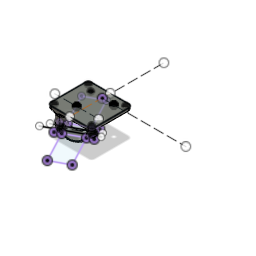
t-echo bracket v3 (Autodesk Fusion 360 design; units mm, degrees)
Autodesk Fusion 360 part; units mm, degrees
note: some values were not read from the file. Chosen so that the rebuilt part matches the saved one: a direction. Set by a fixed rule: which sketch regions a step uses.
sketch "plate" plane through (0, 0, 0) normal (0, 1, 0) x (1, 0, 0)
  line L0 (0, 0) -> (101.1488, 0) construction
  line L1 (0, 0) -> (0, 74.5682) construction
  circle A0 centre (14, 0) radius 1.6
  circle A1 centre (-14, 0) radius 1.6
  line L2 (26, 6) -> (26, -35)
  line L3 (-27, 6) -> (-27, -35)
  line L4 (-23, 10) -> (22, 10)
  line L5 (22, -39) -> (-23, -39)
  arc A2 (-23, 10) -> (-27, 6) centre (-23, 6) ccw
  arc A3 (26, 6) -> (22, 10) centre (22, 6) ccw
  arc A4 (22, -39) -> (26, -35) centre (22, -35) ccw
  arc A5 (-27, -35) -> (-23, -39) centre (-23, -35) ccw
  line L6 (19.5, -24) -> (-33.5, -24) construction
  line L7 (-0.5, -39) -> (-0.5, 10) construction
  point P0 (-7, -24)
  dimension "d1" = 3.2
  dimension "d2" = 14
  dimension "d3" = 12
  dimension "d4" = 53
  dimension "d5" = 10
  dimension "d6" = 39
  dimension "d7" = 4
  dimension "d35" = 20
  dimension "d36" = 15
  constraint coincident L0.start L1.start
  constraint horizontal L0
  constraint perpendicular L0 L1
  constraint coincident L0 A0.centre
  constraint symmetric L1 A0 A1
  constraint vertical L2
  constraint parallel L2 L3
  constraint horizontal L4
  constraint perpendicular L3 L5
  constraint tangent L4 A2
  constraint tangent L3 A2
  constraint tangent L4 A3
  constraint tangent L2 A3
  constraint equal A2 A3
  constraint tangent L2 A4
  constraint tangent L5 A4
  constraint equal A2 A4
  constraint tangent L3 A5
  constraint tangent L5 A5
  constraint equal A2 A5
  constraint midpoint L6 P0
  measures "d1" diameter of A0
  measures "d2" distance of L1 A0.centre
  measures "d3" distance of A0.centre L2
  measures "d4" distance of L2 L3
  measures "d5" distance of A0.centre L4
  measures "d6" distance of A0.centre L5
  measures "d7" radius of A2
  measures "d35" distance of L3 P0
  measures "d36" distance of L5 L6
extrude "Extrude1" add sketch "plate" against normal blind 5 makes body 1
ref_plane "WorkPlane1" through (-6.8327, -2.5, 24.0349) normal (0.469472, 0, 0.882948) x (0, 1, 0)
sketch "bracket" plane through (8.457, 0, 15.9053) normal (0.469472, 0, 0.882948) x (0, 1, 0)
  line L0 (-6, 17.3166) -> (1, 17.3166) construction
  line L1 (-5, 15.6131) -> (-5, -24.1196) construction
  line L2 (-6, 17.3166) -> (-35.5255, 17.3166) construction
  circle A0 centre (-19.15, 17.3166) radius 11.15
  circle A1 centre (-19.15, 17.3166) radius 14.15
  line L3 (-20.15, -0.6834) -> (-18.15, -0.6834)
  line L4 (-18.15, -0.6834) -> (-18.15, 35.3166)
  line L5 (-18.15, 35.3166) -> (-20.15, 35.3166)
  line L6 (-20.15, 35.3166) -> (-20.15, -0.6834)
  line L7 (-20.15, -0.6834) -> (-18.15, 35.3166) construction
  line L8 (-18.15, -0.6834) -> (-20.15, 35.3166) construction
  line L9 (-18.15, -0.6834) -> (-5, -0.6834)
  line L10 (-18.15, 35.3166) -> (-5, 35.3166)
  line L11 (-5, 35.3166) -> (-5, -0.6834)
  line L12 (-20.15, 35.3166) -> (-25.15, 35.3166)
  line L13 (-25.15, 35.3166) -> (-25.15, -0.6834)
  line L14 (-25.15, -0.6834) -> (-20.15, -0.6834)
  point P0 (0, 17.448)
  point P1 (-8, 17.3166)
  point P2 (-19.15, 17.3166)
  dimension "d11" = 22.3
  dimension "d12" = 3
  dimension "d15" = 3
  dimension "d16" = 2
  dimension "d17" = 36
  dimension "d18" = 5
  constraint coincident L0.start L2.start
  constraint parallel L0 L2
  constraint coincident L2 P2
  constraint coincident A0 P1
  constraint coincident L2 P1
  constraint horizontal L3
  constraint perpendicular L3 L4
  constraint parallel L3 L5
  constraint parallel L4 L6
  constraint coincident L7 P2
  constraint coincident L8 P2
  constraint coincident P2 A0.centre
  constraint coincident L1 L9.end
  constraint perpendicular L1 L9
  constraint perpendicular L4 L10
  constraint perpendicular L9 L11
  constraint perpendicular L6 L12
  constraint perpendicular L3 L13
  constraint perpendicular L6 L14
  measures "d11" diameter of A0
  measures "d12" distance of L1 P1
  measures "d16" distance of L4.end L5.end
  measures "d17" distance of L3.end L4.end
  measures "d18" distance of L5.end L12.end
extrude "Extrude2" add sketch "bracket" along normal mid plane 100 separate body contours A0 L4 | A0 L4 L6 | A0 L6 L13 | A0 L13 makes body 2
extrude "Extrude3" add sketch "bracket" along normal mid plane 16 separate body contours A0 A1 L4 | A0 A1 L6 L13 | A1 L4 L10 L11 | A0 A1 L6 L13 | A1 L4 L9 L11 | A0 A1 L13 | A1 L6 L12 L13 | A1 L6 L13 L14 makes body 3 at (4.0897, -21.2398, 21.2476) makes body 4 at (-10.8784, -5, 29.2063)
fillet "Fillet1" radius 5 2 edges at (4.4823, -25.15, 18.0187) (-18.1476, -25.15, 30.0512) on bodies 3
sketch "Sketch3" plane through (0, -25.15, 0) normal (0, -1, 0) x (1, 0, 0)
  line L0 (-24.4291, 24.3305) -> (-16.9176, 38.4577)
  line L1 (-16.9176, 38.4577) -> (-18.9699, 39.549)
  line L2 (-18.9699, 39.549) -> (-26.4815, 25.4218)
  line L3 (-26.4815, 25.4218) -> (-24.4291, 24.3305)
  line L4 (-26.4815, 25.4218) -> (-20.3936, 22.1848)
  line L5 (-20.3936, 22.1848) -> (-0.7832, 11.7578)
  line L6 (-0.7832, 11.7578) -> (5.3046, 8.5208)
  line L7 (-18.9699, 39.549) -> (-26.4815, 25.4218)
  line L8 (-12.8821, 36.312) -> (-18.9699, 39.549)
  line L9 (6.7283, 25.885) -> (-12.8821, 36.312)
  line L10 (12.8162, 22.648) -> (6.7283, 25.885)
  line L11 (5.3046, 8.5208) -> (12.8162, 22.648)
  line L12 (-40.1511, -14.8779) -> (-20.4614, -25.3471)
  line L13 (26.4858, 62.9477) -> (6.7961, 73.4169)
  line L14 (-20.4614, -25.3471) -> (26.4858, 62.9477)
  line L15 (-40.1511, -14.8779) -> (6.7961, 73.4169)
  line L16 (9.0604, 15.5844) -> (-22.7257, 32.4854) construction
  circle A0 centre (-19.3264, 30.6779) radius 3
  circle A1 centre (5.661, 17.3919) radius 3
  circle A2 centre (5.661, 17.3919) radius 1.6
  circle A3 centre (-19.3264, 30.6779) radius 1.6
  line L17 (11.3596, 10.9642) -> (-30.2854, 33.1072)
  line L18 (14.5839, 16.0452) -> (-34.1948, 41.9813)
  dimension "d23" = 6
  dimension "d24" = 6
  dimension "d25" = 3.2
  dimension "d26" = 3.2
  constraint midpoint L11 L16.start
  constraint midpoint L7 L16.end
  constraint coincident L16 A0.centre
  constraint coincident L16 A1.centre
  constraint tangent L14 A1
  constraint tangent L15 A0
  constraint concentric A1 A2
  constraint concentric A0 A3
  constraint parallel L5 L17
  constraint perpendicular L15 L18
  constraint tangent A1 L17
  constraint tangent A0 L18
  measures "d23" diameter of A0
  measures "d24" diameter of A1
  measures "d25" diameter of A2
  measures "d26" diameter of A3
extrude "Extrude4" cut sketch "Sketch3" along normal blind 10 contours L0 A0 A3 | L0 A0 A3 | A1 bodies 3
extrude "Extrude5" cut sketch "Sketch3" along normal mid plane 60 contours L0 A3 | L0 A3 | A2 bodies 3 4
extrude "Extrude7" cut sketch "Sketch3" against normal blind 2.2 from surface at -12 contours L0 L2 L7 A0 L17 L18 | L0 A0 L17 | L0 A0 A3 | L0 A0 A3 | L15 A0 L17 | L0 A0 L18 | L15 A0 L18 | L14 A1 L17 | L14 A1 L18 | A1 | L11 A1 L17 L18 bodies 4
fillet "Fillet2" radius 5 8 edges at (12.8162, -22.65, 22.648) (-26.4815, -22.65, 25.4218) (5.3046, -22.65, 8.5208) (-18.9699, -22.65, 39.549) (12.8162, -11.575, 22.648) (-18.9699, -11.575, 39.549) (-26.4815, -11.575, 25.4218) (5.3046, -11.575, 8.5208) on bodies 3 4
combine "Combine1" operation add target body 4 tool bodies 1
fillet "Fillet3" radius 3 8 edges at (-22.7257, -5, 32.4854) (-24.5009, -5, 26.0273) (-10.5884, -5, 16.9713) (4.6991, -5, 10.5014) (9.0604, -5, 15.5844) (10.8356, -5, 22.0425) (-3.0769, -5, 31.0985) (-18.3644, -5, 37.5684) on bodies 4
fillet "Fillet4" radius 2 16 edges at (-21.382, -26.5319, 22.7104) (-23.1607, -25.3329, 23.8619) (-24.7189, -25.15, 27.4173) (-22.7257, -25.15, 32.4854) (-19.6386, -25.15, 36.9719) (-15.8198, -25.3329, 37.6682) (-13.8705, -26.5319, 36.8375) (-3.0769, -33.3, 31.0985) (7.7167, -26.5319, 25.3594) (9.4954, -25.3329, 24.2079) (11.0536, -25.15, 20.6526) (9.0604, -25.15, 15.5844) (5.9733, -25.15, 11.0979) (2.1545, -25.3329, 10.4016) (0.2052, -26.5319, 11.2323) (-10.5884, -33.3, 16.9713) on bodies 3
fillet "Fillet5" radius 2 13 edges at (5.2263, -5, 39) (-12.587, -5.04, 39) (-17.7534, -5.5467, 39) (-22.4711, -5, 39) (-25.8284, -5, 37.8284) (-27, -5, 32.9024) (-27, -5.0875, 27.4892) (-27, -5, 9.0868) (-25.8284, -5, -8.8284) (-0.5, -5, -10) (24.8284, -5, -8.8284) (26, -5, 14.5) (24.8284, -5, 37.8284) on bodies 4
hidden bodies 2
equation "d10 = ( 90 deg - 62 deg )"
named bodies: "base", "tube", "t-echo clamp top", "t-echo clamp base"
